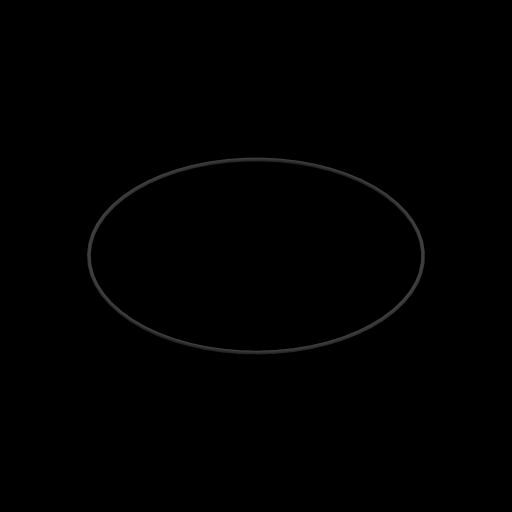
# Autodesk Inventor part: OringV2
Saved by Autodesk Inventor 2024 (Build 280153000, 153)
## iProperties
Created: 2026-04-12
Part Number: OringV2
Material: Generic
Document SubType Name: Modeling
Designer: Tanner
Density: 1 g/cm^3
Appearance: Rubber - Black
Author: Tanner
Autodesk Inventor part; units mm, degrees
ref_plane "YZ Plane" through (0, 0, 0) normal (1, 0, 0) x (0, 1, 0)
ref_plane "XZ Plane" through (0, 0, 0) normal (0, 1, 0) x (-1, 0, 0)
ref_plane "XY Plane" through (0, 0, 0) normal (0, 0, 1) x (1, 0, 0)
sketch "Sketch1" plane through (0, 0, 0) normal (0, 0, 1) x (1, 0, 0)
  line L0 (-103.9813, 2.3813) -> (-101.6, 2.3813) construction
  line L1 (-101.6, 2.3813) -> (-101.6, 0) construction
  line L2 (-101.6, 0) -> (-103.9813, 0) construction
  line L3 (-103.9813, 0) -> (-103.9813, 2.3813) construction
  line L4 (-103.9813, 2.3813) -> (-101.6, 0) construction
  line L5 (-101.6, 2.3813) -> (-103.9813, 0) construction
  circle A0 centre (-102.7906, 1.1906) radius 1.1906
  line L6 (0, -0.4763) -> (0, 2.8575) projected
  point P0 (0, 0)
  dimension "d0" = 2.3813
  dimension "d1" = 2.3813
  dimension "d2" = 101.6
  constraints: 12 end point, 2 midpoint, 2 parallel, 1 centre point, 1 coincident, 1 horizontal, 1 horizontal alignment, 1 perpendicular, 1 tangent
  measures "d0" distance of L1.end L2.end
  measures "d1" distance of L0.end L1.end
  measures "d2" distance from line of point (0, 0) L1
revolve "Revolution1" add sketch "Sketch1" angle 360 about axis through (0, -10, 0) along (0, 1, 0)
body "Solid1"
